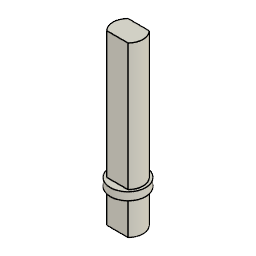
Drive_Wheel_Ax (Autodesk Fusion 360 design; units mm, degrees)
Autodesk Fusion 360 part; units mm, degrees
sketch "Wheel_Ax_Sketch" plane through (0, 0, 0) normal (0, 0, 1) x (1, 0, 0)
  arc A0 (-3, 3) -> (-3, -3) centre (0, 0) ccw
  arc A1 (-3, 3) -> (-3, -3) centre (0, 0) ccw
  line L0 (-3, -3) -> (3, -3)
  arc A2 (3, -3) -> (3, 3) centre (0, 0) ccw
  line L1 (3, 3) -> (-3, 3)
  circle A3 centre (0, 0) radius 5
  dimension "d1" = 10
  constraint concentric A1 A3
  measures "d1" diameter of A3
extrude "Extrude1" add sketch "Wheel_Ax_Sketch" along normal blind 47.5 contours A0 A1 L0 A2 L1
extrude "Extrude2" add sketch "Wheel_Ax_Sketch" along normal blind 2.2 from surface at 9.5
named bodies: "Wheel_Ax_Body"
